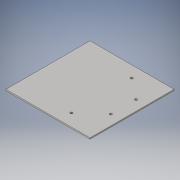
# Autodesk Inventor part: side panel v1.2
Saved by Autodesk Inventor 2016 (Build 200138000, 138)
## iProperties
Created: 2015-10-10
Part Number: side panel v1.2
Material: Generic
Document SubType Name: Modeling
Designer: Delta
Density: 1 g/cm^3
Appearance: Default
Author: Delta
Autodesk Inventor part; units mm, degrees
ref_plane "YZ Plane" through (0, 0, 0) normal (1, 0, 0) x (0, 1, 0)
ref_plane "XZ Plane" through (0, 0, 0) normal (0, 1, 0) x (-1, 0, 0)
ref_plane "XY Plane" through (0, 0, 0) normal (0, 0, 1) x (1, 0, 0)
sketch "Sketch1" plane through (0, 0, 0) normal (0, 1, 0) x (-1, 0, 0)
  line L0 (0, 0) -> (215.9, 0)
  line L1 (215.9, 0) -> (215.9, -215.9)
  line L2 (215.9, -215.9) -> (0, -215.9)
  line L3 (0, -215.9) -> (0, 0)
  dimension "d0" = 215.9
  dimension "d1" = 215.9
  constraints: 8 end point, 2 parallel, 1 horizontal, 1 perpendicular
  measures "d0" distance of L1.end L2.end
  measures "d1" distance of L0.end L1.end
extrude "Extrusion1" add sketch "Sketch1" along normal blind 3.175
sketch "Sketch2" plane through (0, 3.175, 0) normal (0, 1, 0) x (1, 0, 0)
  line L0 (-291.9068, 6.35) -> (0, 6.35)
  line L1 (0, 6.35) -> (0, 293.5185)
  line L2 (0, 293.5185) -> (-291.9068, 293.5185)
  line L3 (-291.9068, 293.5185) -> (-291.9068, 6.35)
  line L4 (-215.9, 0) -> (0, 0) projected
  line L5 (0, 0) -> (0, 215.9) projected
  point P0 (-26, 79.35)
  point P1 (-79, 31.35)
  point P2 (-79, 186.35)
  point P3 (-26, 144.35)
  dimension "d4" = 138
  dimension "d5" = 26
  dimension "d6" = 79
  dimension "d7" = 25
  dimension "d8" = 79
  dimension "d9" = 26
  dimension "d10" = 73
  dimension "d11" = 180
  dimension "d12" = 6.35
  dimension "d13" = 0
  constraints: 8 end point
  measures "d4" distance from line of L0 point (-26, 144.35)
  measures "d5" distance from line of L1 point (-26, 144.35)
  measures "d6" distance from line of L1 point (-79, 186.35)
  measures "d7" distance from line of L0 point (-79, 31.35)
  measures "d8" distance from line of L1 point (-79, 31.35)
  measures "d9" distance from line of L1 point (-26, 79.35)
  measures "d10" distance from line of L0 point (-26, 79.35)
  measures "d11" distance from line of L0 point (-79, 186.35)
  measures "d12" distance between parallel lines of L4 L0
  measures "d13" distance between parallel lines of L5 L1
hole "Hole1" at (-26, 3.175, -79.35) at (-79, 3.175, -31.35) at (-79, 3.175, -186.35) at (-26, 3.175, -144.35) direction (0, -1, 0) diameter 6 end through all
body "Solid1"
